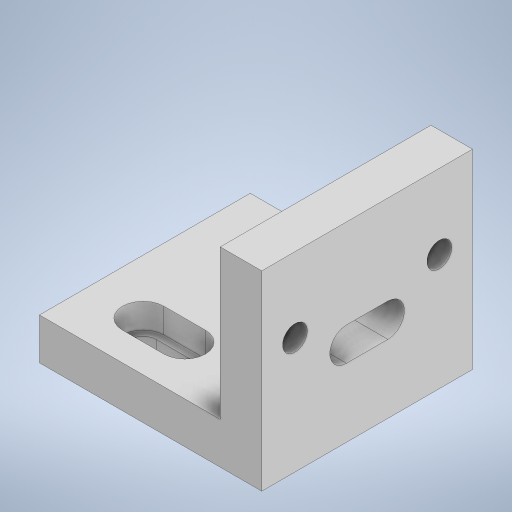
# Autodesk Inventor part: Actuator Stage End Cap
Saved by Autodesk Inventor 2024 (Build 280153000, 153)
## iProperties
Created: 2024-10-16
Part Number: Actuator Stage End Cap
Material: Generic
Document SubType Name: Modeling
Designer: Kemper Room 121
Density: 1 g/cm^3
Appearance: Default
Author: Kemper Room 121
Autodesk Inventor part; units mm, degrees
ref_plane "YZ Plane" through (0, 0, 0) normal (1, 0, 0) x (0, 1, 0)
ref_plane "XZ Plane" through (0, 0, 0) normal (0, 1, 0) x (-1, 0, 0)
ref_plane "XY Plane" through (0, 0, 0) normal (0, 0, 1) x (1, 0, 0)
sketch "Sketch1" plane through (0, 0, 0) normal (0, 1, 0) x (-1, 0, 0)
  line L0 (0, 0) -> (53.575, 0)
  line L1 (53.575, 0) -> (53.575, -50.8)
  line L2 (53.575, -50.8) -> (0, -50.8)
  line L3 (0, -50.8) -> (0, 0)
  line L4 (10, 0) -> (10, -50.8)
  arc A0 (30.4, -35.8017) -> (30.4, -42.1517) centre (30.4, -38.9767) ccw
  arc A1 (40.4, -42.1517) -> (40.4, -35.8017) centre (40.4, -38.9767) ccw
  line L5 (30.4, -35.8017) -> (40.4, -35.8017)
  line L6 (40.4, -42.1517) -> (30.4, -42.1517)
  line L7 (-7.5059, -25.4) -> (68.7329, -25.4)
  arc A2 (30.4, -8.6483) -> (30.4, -14.9983) centre (30.4, -11.8233) ccw
  arc A3 (40.4, -14.9983) -> (40.4, -8.6483) centre (40.4, -11.8233) ccw
  line L8 (30.4, -14.9983) -> (40.4, -14.9983)
  line L9 (40.4, -8.6483) -> (30.4, -8.6483)
  dimension "d0" = 50.8
  dimension "d2" = 10
  dimension "d3" = 6.35
  dimension "d4" = 6.35
  dimension "d6" = 10
  dimension "d7" = 20.4
  dimension "d8" = 13.175
  dimension "d9" = 25.4
  constraints: 20 end point, 8 point on circle, 6 symmetric about line, 4 centre point, 3 tangent, 2 horizontal, 2 parallel, 2 perpendicular, 2 point on line, 2 other
  measures "d0" distance of L2.end L0.start
  measures "d2" distance between parallel lines of L3 L4
  measures "d3" diameter of A0
  measures "d4" diameter of A1
  measures "d6" distance of L6.start L6.end
  measures "d7" distance from line of L4 A0.centre
  measures "d8" distance from line of L1 A1.centre
  measures "d9" distance between parallel lines of L0 L7
extrude "Extrusion1" add sketch "Sketch1" along normal blind 10
sketch "Sketch2" plane through (0, 10, 0) normal (0, 1, 0) x (1, 0, 0)
  line L0 (0, 50.8) -> (-53.575, 50.8) projected
  line L1 (0, 0) -> (-10, 0)
  line L2 (-10, 0) -> (-10, 50.8)
  line L3 (-10, 50.8) -> (0, 50.8)
  line L4 (0, 50.8) -> (0, 0)
  dimension "d12" = 10
  constraints: 8 end point, 2 parallel, 1 horizontal, 1 perpendicular, 1 point on line
  measures "d12" distance between parallel lines of L4 L2
extrude "Extrusion2" add sketch "Sketch2" along normal blind 36
sketch "Sketch3" plane through (0, 0, 0) normal (1, 0, 0) x (0, 0, -1)
  line L0 (0, 10) -> (50.8, 10) projected
  circle A0 centre (8, 28) radius 1.42
  circle A1 centre (42.8, 28) radius 1.42
  line L1 (50.8, 0) -> (50.8, 46) projected
  line L2 (0, 0) -> (0, 46) projected
  line L3 (0, 0) -> (50.8, 0) projected
  line L4 (50.8, 0) -> (50.8, 46) projected
  line L5 (0, 46) -> (50.8, 46) projected
  line L6 (0, 0) -> (0, 46) projected
  arc A2 (20.4, 24.5) -> (20.4, 16.5) centre (20.4, 20.5) ccw
  arc A3 (30.4, 16.5) -> (30.4, 24.5) centre (30.4, 20.5) ccw
  line L7 (20.4, 24.5) -> (30.4, 24.5)
  line L8 (20.4, 16.5) -> (30.4, 16.5)
  line L9 (20.4, 20.5) -> (25.4, 20.5)
  point P0 (50.8, 23)
  point P1 (25.4, 10)
  dimension "d15" = 2.84
  dimension "d16" = 2.84
  dimension "d17" = 34.8
  dimension "d18" = 0
  dimension "d19" = 18
  dimension "d20" = 8
  dimension "d21" = 8
  dimension "d22" = 50.8
  dimension "d35" = 8
  dimension "d36" = 8
  dimension "d37" = 0
  dimension "d38" = 10
  dimension "d39" = 5
  dimension "d40" = 25.4
  dimension "d41" = 10.5
  constraints: 6 end point, 4 centre point, 4 point on circle, 2 midpoint, 2 tangent, 1 horizontal
  measures "d15" diameter of A0
  measures "d16" diameter of A1
  measures "d17" distance of A0.centre A1.centre
  measures "d18" vertical distance of A0.centre A1.centre
  measures "d19" distance from line of L0 A1.centre
  measures "d20" distance from line of L1 A1.centre
  measures "d21" distance from line of L2 A0.centre
  measures "d22" distance of L5.start L4.end
  measures "d35" diameter of A2
  measures "d36" diameter of A3
  measures "d37" vertical distance of L9.start A3.centre
  measures "d38" distance of L9.start A3.centre
  measures "d39" distance of L9.start L9.end
  measures "d40" horizontal distance of point (50.8, 23) L9.end
  measures "d41" distance of point (25.4, 10) L9.end
extrude "Extrusion3" cut sketch "Sketch3" against normal blind 36 contours A0 | A1 | L7 A3 L8 A2
sketch "Sketch4" plane through (0, 10, 0) normal (0, 1, 0) x (1, 0, 0)
  arc A0 (-40.4, 42.1517) -> (-40.4, 35.8017) centre (-40.4, 38.9767) ccw projected
  arc A1 (-40.4, 43.9767) -> (-40.4, 33.9767) centre (-40.4, 38.9767) ccw
  arc A2 (-30.4, 35.8017) -> (-30.4, 42.1517) centre (-30.4, 38.9767) ccw projected
  arc A3 (-30.4, 33.9767) -> (-30.4, 43.9767) centre (-30.4, 38.9767) ccw
  line L0 (-10, 0) -> (-10, 50.8) projected
  line L1 (-10, 50.8) -> (-53.575, 50.8) projected
  line L2 (-53.575, 50.8) -> (-53.575, 0) projected
  line L3 (-53.575, 0) -> (-10, 0) projected
  line L4 (-40.4, 14.9983) -> (-30.4, 14.9983) projected
  arc A4 (-30.4, 8.6483) -> (-30.4, 14.9983) centre (-30.4, 11.8233) ccw projected
  line L5 (-30.4, 8.6483) -> (-40.4, 8.6483) projected
  arc A5 (-40.4, 14.9983) -> (-40.4, 8.6483) centre (-40.4, 11.8233) ccw projected
  line L6 (-40.4, 42.1517) -> (-30.4, 42.1517) projected
  arc A6 (-30.4, 35.8017) -> (-30.4, 42.1517) centre (-30.4, 38.9767) ccw projected
  line L7 (-30.4, 35.8017) -> (-40.4, 35.8017) projected
  arc A7 (-40.4, 42.1517) -> (-40.4, 35.8017) centre (-40.4, 38.9767) ccw projected
  arc A8 (-40.4, 16.8233) -> (-40.4, 6.8233) centre (-40.4, 11.8233) ccw
  arc A9 (-30.4, 6.8233) -> (-30.4, 16.8233) centre (-30.4, 11.8233) ccw
  line L8 (-30.4, 6.8233) -> (-40.4, 6.8233)
  line L9 (-40.4, 16.8233) -> (-30.4, 16.8233)
  line L10 (-30.4, 33.9767) -> (-40.4, 33.9767)
  line L11 (-40.4, 43.9767) -> (-30.4, 43.9767)
  point P0 (0, 0)
  dimension "d25" = 10
  dimension "d26" = 10
  dimension "d27" = 10
  dimension "d28" = 10
  constraints: 8 end point, 8 point on circle, 5 tangent, 4 centre point, 4 coincident, 2 parallel
  measures "d25" diameter of A1
  measures "d26" diameter of A3
  measures "d27" diameter of A8
  measures "d28" diameter of A9
extrude "Extrusion4" cut sketch "Sketch4" against normal blind 6 contours L6 A2 L7 A0 | L11 A3 L10 A1 | L4 A4 L5 A5 | L9 A9 L8 A8
sketch "Sketch5" plane through (0, 0, 0) normal (1, 0, 0) x (0, 0, -1)
  circle A0 centre (42.8, 28) radius 1.42 projected
  circle A1 centre (8, 28) radius 1.42 projected
  line L0 (0, 0) -> (50.8, 0) projected
  line L1 (50.8, 0) -> (50.8, 46) projected
  line L2 (0, 46) -> (50.8, 46) projected
  line L3 (0, 0) -> (0, 46) projected
  circle A2 centre (8, 28) radius 3
  circle A3 centre (42.8, 28) radius 1.42 projected
  circle A4 centre (42.8, 28) radius 3
  dimension "d31" = 6
  dimension "d32" = 6
  constraints: 2 centre point, 2 coincident
  measures "d31" diameter of A2
  measures "d32" diameter of A4
extrude "Extrusion5" cut sketch "Sketch5" against normal blind 5 contours A1 | A2 | A4
equation "\"d4\" = d3"
equation "\"d9\" = 0.5 * d0"
equation "\"d12\" = d2"
equation "\"d16\" = d15"
equation "\"d20\" = -0.5 * d17 + 0.5 * d22"
equation "\"d36\" = d35"
equation "\"d39\" = 0.5 * d38"
equation "\"d40\" = 0.5 * d22"
equation "\"d26\" = d25"
equation "\"d27\" = d25"
equation "\"d28\" = d25"
equation "\"d32\" = d31"
body "Solid1"
